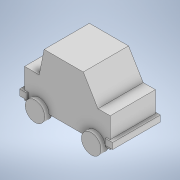
# Autodesk Inventor part: Car
Saved by Autodesk Inventor 2021 (Build 250183000, 183)
## iProperties
Created: 2021-08-08
Part Number: Car
Material: Generic
Document SubType Name: Modeling
Designer: Shammy Haider
Density: 1 g/cm^3
Appearance: Default
Author: Shammy Haider
Autodesk Inventor part; units mm, degrees
ref_plane "YZ Plane" through (0, 0, 0) normal (1, 0, 0) x (0, 1, 0)
sketch "Sketch1" plane through (0, 0, 0) normal (0, 0, 1) x (1, 0, 0)
  line L0 (17.5, -6) -> (-17.5, -6)
  line L1 (-17.5, -6) -> (-17.5, 6)
  line L2 (-17.5, 6) -> (17.5, 6)
  line L3 (17.5, 6) -> (17.5, -6)
  line L4 (17.5, -6) -> (-17.5, 6) construction
  line L5 (-17.5, -6) -> (17.5, 6) construction
  line L6 (-11.5, 6) -> (-9.5, 16)
  line L7 (-9.5, 16) -> (6.5, 16)
  line L8 (6.5, 16) -> (12.5, 6)
  point P0 (0, 0)
  dimension "d0" = 35
  dimension "d1" = 12
  dimension "d2" = 16
  dimension "d3" = 6
  dimension "d4" = 5
  dimension "d5" = 11
  dimension "d6" = 16
  constraints: 18 end point, 2 horizontal, 2 midpoint, 2 parallel, 2 point on line, 1 perpendicular
  measures "d0" distance of L1.end L2.end
  measures "d1" distance of L0.end L1.end
  measures "d2" distance of L6.end L7.end
  measures "d3" distance of L1.end L6.start
  measures "d4" distance of L2.end L8.end
  measures "d5" horizontal distance of L2.end L7.end
  measures "d6" distance from line of point (0, 0) L7
extrude "Extrusion1" add sketch "Sketch1" along normal mid plane 18.5
sketch "Sketch2" plane through (0, 0, 0) normal (0, 0, 1) x (1, 0, 0)
  line L0 (17.5, -6) -> (-17.5, -6) projected
  circle A0 centre (-11.5, -6) radius 4
  circle A1 centre (11.5, -6) radius 4
  line L1 (17.5, -6) -> (17.5, 6) projected
  point P0 (0, 0)
  dimension "d9" = 8
  dimension "d10" = 8
  dimension "d11" = 6
  dimension "d12" = 23
  constraints: 2 centre point, 2 point on line
  measures "d9" diameter of A0
  measures "d10" diameter of A1
  measures "d11" distance from line of L1 A1.centre
  measures "d12" distance of A1.centre A0.centre
extrude "Extrusion2" add sketch "Sketch2" along normal mid plane 22
sketch "Sketch3" plane through (-17.5, -6, 9.25) normal (-1, 0, 0) x (0, 0, 1)
  line L0 (-17.25, 0) -> (-1.25, 0)
  line L1 (-1.25, 0) -> (-1.25, -5.8773)
  line L2 (-1.25, -5.8773) -> (-17.25, -5.8773)
  line L3 (-17.25, -5.8773) -> (-17.25, 0)
  line L4 (1.75, -4) -> (1.75, 4) projected
  line L5 (0, 0) -> (-18.5, 0) projected
  point P0 (-9.25, 6)
  dimension "d15" = 16
  dimension "d16" = 3
  constraints: 8 end point, 2 parallel, 1 collinear, 1 horizontal, 1 perpendicular
  measures "d15" distance of L1.end L2.end
  measures "d16" distance between parallel lines of L4 L1
extrude "Extrusion3" cut sketch "Sketch3" against normal blind 35
ref_plane "Work Plane1" through (-19, -6, 9.25) normal (-1, 0, 0) x (0, 0, 1)
sketch "Sketch4" plane through (-19, -6, 9.25) normal (-1, 0, 0) x (0, 0, 1)
  line L0 (-19, 3.5348) -> (0.5, 3.5348)
  line L1 (0.5, 3.5348) -> (0.5, 1.0348)
  line L2 (0.5, 1.0348) -> (-19, 1.0348)
  line L3 (-19, 1.0348) -> (-19, 3.5348)
  line L4 (0, 12) -> (0, 0) projected
  point P0 (-9.25, 6)
  dimension "d20" = 2.5
  dimension "d21" = 19.5
  dimension "d22" = 0.5
  constraints: 8 end point, 2 parallel, 1 horizontal, 1 perpendicular
  measures "d20" distance of L0.end L1.end
  measures "d21" distance of L0.start L0.end
  measures "d22" distance between parallel lines of L1 L4
extrude "Extrusion4" add sketch "Sketch4" against normal blind 3
mirror "Mirror1" about plane through (0, 0, 0) normal (1, 0, 0) of "Extrusion4"
ref_plane "Work Plane3" through (5.5, 6, 9.25) normal (1, 0, 0) x (0, 0, -1)
sketch "Sketch5" plane through (5.5, 6, 9.25) normal (1, 0, 0) x (0, 0, -1)
  line L0 (1.25, -16) -> (-1.75, -16) projected
  line L1 (20.25, -16) -> (17.25, -16) projected
  circle A0 centre (9.25, -16) radius 2.5
  point P0 (9.25, -6)
  dimension "d26" = 5
  constraints: 1 centre point, 1 coincident
  measures "d26" diameter of A0
boundary_patch "Boundary Patch1"
body "Solid1"
body "Srf1"
